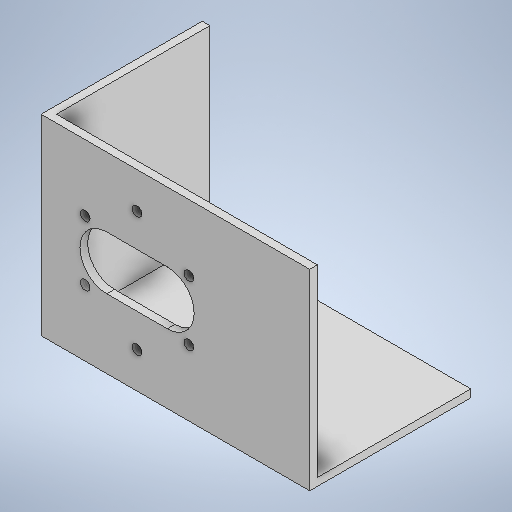
# Autodesk Inventor part: extendeddrivemotorcasing
Saved by Autodesk Inventor 2025.2 (Build 292293000, 293)
## iProperties
Created: 2026-03-25
Part Number: extendeddrivemotorcasing
Material: Generic
Document SubType Name: Modeling
Designer: hp
Density: 1 g/cm^3
Appearance: Default
Author: hp
Autodesk Inventor part; units mm, degrees
ref_plane "YZ Plane" through (0, 0, 0) normal (1, 0, 0) x (0, 1, 0)
ref_plane "XZ Plane" through (0, 0, 0) normal (0, 1, 0) x (-1, 0, 0)
ref_plane "XY Plane" through (0, 0, 0) normal (0, 0, 1) x (1, 0, 0)
sketch "Sketch1" plane through (0, 0, 0) normal (0, 0, 1) x (1, 0, 0)
  circle A0 centre (0, 0) radius 18.38
  circle A1 centre (13.5143, 7.8025) radius 1.255
  circle A2 centre (0, 15.605) radius 1.255
  circle A3 centre (-13.5143, 7.8025) radius 1.255
  circle A4 centre (-13.5143, -7.8025) radius 1.255
  circle A5 centre (0, -15.605) radius 1.255
  circle A6 centre (13.5143, -7.8025) radius 1.255
  circle A7 centre (7.9, 0) radius 5.98
  line L0 (25, 25) -> (-25, 25)
  line L1 (-25, 25) -> (-25, -25)
  line L2 (-25, -25) -> (25, -25)
  line L3 (25, -25) -> (25, 25)
  line L4 (25, 25) -> (-25, -25) construction
  line L5 (-25, 25) -> (25, -25) construction
  circle A8 centre (7.9, 0) radius 6.98
  line L6 (7.9, -6.98) -> (-7.9, -6.98)
  line L7 (7.9, 6.98) -> (-7.9, 6.98)
  circle A9 centre (-7.9, 0) radius 6.98
  line L8 (23, 23) -> (-23, 23)
  line L9 (-23, 23) -> (-23, -23)
  line L10 (-23, -23) -> (23, -23)
  line L11 (23, -23) -> (23, 23)
  line L12 (-23, 23) -> (-23, 25)
  line L13 (23, 23) -> (23, 25)
  line L14 (23, -23) -> (23, -25)
  line L15 (23, -23) -> (25, -23)
  point P0 (0, 0)
  dimension "d0" = 50
  dimension "d1" = 50
  dimension "d2" = 1
  dimension "d3" = 15.8
  dimension "d6" = 2
  constraints: 32 end point, 9 centre point, 5 perpendicular, 5 point on line, 4 parallel, 3 horizontal, 2 coincident, 2 midpoint, 2 point on circle, 2 tangent, 6 other
  measures "d0" distance of L2.end L1.end
  measures "d1" distance of L1.end L0.end
  measures "d2" radial gap between concentric circles of A7 A8
  measures "d3" distance of L6.start L6.end
  measures "d6" distance between parallel lines of L3 L11
extrude "Extrusion1" add sketch "Sketch1" along normal blind 2 contours A0 | L3 L15 L11 L13 L0 | L13 L8 L12 L0 | L3 L2 L14 L15 | L12 L9 L10 L14 L2 L1 L0 | L11 L10 L9 L8
extrude "Extrusion2" add sketch "Sketch1" against normal blind 40 contours L3 L2 L14 L15 | L12 L9 L10 L14 L2 L1 L0
thread "Thread1" size "M2.5x0.45" class "6H" standard "ISO Metric profile" length 10
thread "Thread2" size "M2.5x0.45" class "6H" standard "ANSI Metric M Profile" length 10
thread "Thread3" size "M2.5x0.45" class "6H" standard "ISO Metric profile" full length
thread "Thread4" size "M2.5x0.45" class "6H" standard "ANSI Metric M Profile" full length
thread "Thread5" size "M2.5x0.45" class "6H" standard "ANSI Metric M Profile" full length
thread "Thread6" size "M2.5x0.45" class "6H" standard "ANSI Metric M Profile" full length
sketch "Sketch2" plane through (25, -25, 0) normal (1, 0, 0) x (0, 0, -1)
  line L0 (0, 2) -> (0, 50) projected
  line L1 (0, 2) -> (40, 2) projected
  line L2 (40, 2) -> (40, 0) projected
  line L3 (0, 0) -> (40, 0) projected
  line L4 (40, 0) -> (-2, 0) projected
  line L5 (-2, 0) -> (-2, 50) projected
  line L6 (0, 50) -> (-2, 50) projected
  point P0 (0, 25)
extrude "Extrusion3" add sketch "Sketch2" along normal blind 20
body "Solid1"
